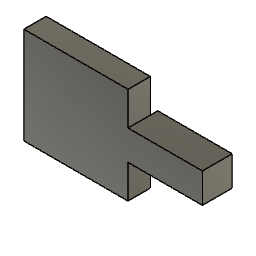
ppp3 v4 (Autodesk Fusion 360 design; units mm, degrees)
Autodesk Fusion 360 part; units mm, degrees
sketch "Sketch1" plane through (0, 0, 0) normal (0, 1, 0) x (1, 0, 0)
  line L0 (0, 0) -> (-14, 0)
  line L1 (-14, 0) -> (-14, -13)
  line L2 (-14, -13) -> (0, -13)
  line L3 (0, -13) -> (0, 0)
  constraint horizontal L0
  constraint vertical L1
  constraint horizontal L2
  constraint vertical L3
  constraint coincident L0.start L3.end
extrude "Extrude1" add sketch "Sketch1" along normal blind 3
sketch "Sketch2" plane through (0, 0, 0) normal (0, 1, 0) x (1, 0, 0)
  line L0 (0, -8.5) -> (20, -8.5)
  line L1 (20, -8.5) -> (20, -4.5)
  line L2 (20, -4.5) -> (0, -4.5)
  line L3 (0, -4.5) -> (0, -8.5)
  point P0 (0, -13)
  dimension "d3" = 4
  dimension "d4" = 4.5
  constraint horizontal L0
  constraint vertical L1
  constraint horizontal L2
  constraint vertical L3
  measures "d3" distance of L0.end L1.end
  measures "d4" distance of L0.start P0
extrude "Extrude2" add sketch "Sketch2" along normal blind 8
delete_face "DeleteFace1" 1 faces at (13.3333, 3.6667, 8.5)
sketch "Sketch3" plane through (0, 0, 0) normal (0, 1, 0) x (1, 0, 0)
  line L0 (0, -8.5) -> (10, -8.5)
  line L1 (10, -8.5) -> (10, -4.5)
  line L2 (10, -4.5) -> (0, -4.5)
  line L3 (0, -4.5) -> (0, -8.5)
  dimension "d7" = 10
  dimension "d8" = 4.5
  constraint horizontal L0
  constraint vertical L1
  constraint horizontal L2
  constraint vertical L3
  measures "d7" distance of L0.start L0.end
  measures "d8" distance of origin L2.end
extrude "Extrude3" add sketch "Sketch3" along normal blind 4
